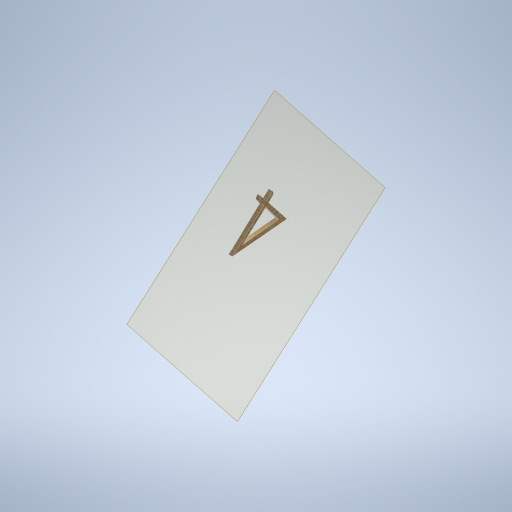
# Autodesk Inventor part: panel_block_03
Saved by Autodesk Inventor 2024.2 (Build 282272000, 272)
## iProperties
Created: 2024-05-21
Part Number: panel_block_03
Material: Wood (Maple)
Document SubType Name: Modeling
Designer: LOSTER_1
Density: 0.67 g/cm^3
Appearance: Natural Maple - Glossy Dark Tint
Author: LOSTER_1
Autodesk Inventor part; units mm, degrees
ref_plane "XZ Plane" through (0, 0, 0) normal (0, 1, 0) x (-1, 0, 0)
sketch "Sketch1" plane through (0, 0, 0) normal (0, 0, 1) x (1, 0, 0)
  arc A0 (4796.3585, -1909.6289) -> (3343.4744, 1121.5056) centre (-3903.1767, -4215.7265) ccw
  line L0 (3236.8192, 1046.7661) -> (3343.5051, 1121.464)
  arc A1 (3228.7635, 1285.3391) -> (1546.1726, 3076.3751) centre (-4110.5601, -3923.7232) ccw
  line L1 (3228.7635, 1285.3391) -> (3122.0787, 1210.6419)
  line L2 (1372.9503, 3176.3452) -> (1308.1705, 3064.1503)
  arc A2 (1372.9503, 3176.3452) -> (93.8576, 4024.2684) centre (-4221.2651, -3873.8147) ccw
  line L3 (1481.3729, 2964.1457) -> (1546.1726, 3076.3751)
  arc A3 (4543.4821, -2147.4888) -> (93.8528, 3844.2289) centre (-4256.4671, -4034.5221) ccw
  line L4 (93.8576, 4024.2684) -> (93.8528, 3844.2289)
  line L5 (1308.1705, 3064.1503) -> (1481.3729, 2964.1457)
  line L6 (3122.0787, 1210.6419) -> (3236.8192, 1046.7661)
  arc A4 (4543.4821, -2147.4888) -> (4796.3585, -1909.6289) centre (4134.8595, -1459.7188) ccw
  point P0 (0, 0)
  dimension "d7" = 800
  constraints: 14 end point, 11 point on circle, 5 centre point, 1 perpendicular
  measures "d7" radius of A4
ref_plane "Work Plane2" through (0, 0, -8101) normal (0, 0, 1) x (1, 0, 0)
ref_plane "Work Plane1" through (0, 0, 0) normal (0, 0, 1) x (1, 0, 0)
sketch "Sketch2" plane through (0, 0, -8101) normal (0, 0, 1) x (1, 0, 0)
  arc A0 (1192.0552, 3508.338) -> (93.8528, 4294.485) centre (-5164.5547, -4211.3454) ccw projected
  arc A1 (3133.8513, 1483.0798) -> (1365.2603, 3408.338) centre (-5051.6105, -4261.3276) ccw projected
  arc A2 (4543.6426, -2147.8414) -> (93.8528, 4114.0508) centre (-5207.4444, -4365.1147) ccw projected
  line L0 (1192.0552, 3508.338) -> (1126.9741, 3395.6142) projected
  line L1 (1365.2603, 3408.338) -> (1300.1792, 3295.6142) projected
  line L2 (1126.9741, 3395.6142) -> (1300.1792, 3295.6142) projected
  line L3 (93.8528, 4294.485) -> (93.8528, 4114.0508) projected
  line L4 (3027.6129, 1408.6909) -> (3133.8513, 1483.0798) projected
  line L5 (3142.3282, 1244.8605) -> (3248.5665, 1319.2494) projected
  line L6 (3027.6129, 1408.6909) -> (3142.3282, 1244.8605) projected
  arc A3 (4803.6655, -1899.2732) -> (3248.5665, 1319.2494) centre (-4832.968, -4570.4704) ccw projected
  arc A4 (4543.6426, -2147.8414) -> (4803.6655, -1899.2732) centre (4135.0016, -1460.0824) ccw projected
  point P0 (0, 0)
loft "Loft1" add profiles "Sketch1", "Sketch2"
ref_plane "Work Plane3" through (2600, 0, 0) normal (1, 0, 0) x (0, 1, 0)
sketch "Sketch3" plane through (2600, 0, 0) normal (1, 0, 0) x (0, 1, 0)
  line L0 (3120.8038, -3828.6818) -> (2179.9067, -2717.5683)
  line L1 (2179.9067, -2717.5683) -> (2281.1646, -4539.693)
  line L2 (2281.1646, -4539.693) -> (3120.8038, -3828.6818)
  line L3 (4534.6211, 332.5956) -> (-2270.5383, 332.5956)
  line L4 (-2270.5383, 332.5956) -> (-2270.5383, -8394.1003)
  line L5 (-2270.5383, -8394.1003) -> (4534.6211, -8394.1003)
  line L6 (4534.6211, -8394.1003) -> (4534.6211, 332.5956)
  point P0 (0, 0)
  constraints: 14 end point, 2 parallel, 2 perpendicular, 1 horizontal
extrude "Extrusion1" cut sketch "Sketch3" along normal through all both and the other way through all
sketch "Sketch5" plane through (2219.0112, 2281.1646, -4539.693) normal (0, -0.9984595, -0.0554857) x (1, 0, 0)
  line L0 (318.8718, 1824.936) -> (250.4195, 0)
  point P0 (-2219.0112, 4659.2715)
  constraints: 2 end point, 1 other
ref_plane "Work Plane4" through (2537.8831, 2179.9067, -2717.5683) normal (-0.6423359, -0.7662012, -0.0184479) x (-0.0374831, 0.0554467, -0.9977578)
sketch "Sketch6" plane through (2537.8831, 2179.9067, -2717.5683) normal (-0.6423359, -0.7662012, -0.0184479) x (-0.0374831, 0.0554467, -0.9977578)
  line L0 (-729.0595, -1938.3665) -> (2085.591, -1938.3665)
  line L1 (2085.591, -1938.3665) -> (2085.591, 179.9667)
  line L2 (2085.591, 179.9667) -> (-729.0595, 179.9667)
  line L3 (-729.0595, 179.9667) -> (-729.0595, -1938.3665)
  point P0 (-2737.216, -722.0143)
  constraints: 8 end point, 2 parallel, 1 horizontal, 1 perpendicular
extrude "Extrusion2" cut sketch "Sketch6" against normal through all
ref_plane "Work Plane5" through (2537.8831, 2179.9067, -2717.5683) normal (-0.9992973, -0.0020798, 0.0374254) x (-0.0374831, 0.0554467, -0.9977578)
sketch "Sketch7" plane through (2537.8831, 2179.9067, -2717.5683) normal (-0.9992973, -0.0020798, 0.0374254) x (-0.0374831, 0.0554467, -0.9977578)
  line L0 (1826.2193, 0) -> (0, 0) projected
  line L1 (1201.6643, -877.7967) -> (1826.2193, 0) projected
  line L2 (0, 0) -> (1201.6643, -877.7967) projected
  point P0 (-2737.216, 2025.7624)
sketch "Sketch8" plane through (2537.8831, 2179.9067, -2717.5683) normal (-0.6423359, -0.7662012, -0.0184479) x (-0.0374831, 0.0554467, -0.9977578)
  line L0 (1826.2193, 0) -> (0, 0) projected
  line L1 (1201.6643, -1365.6093) -> (1826.2193, 0) projected
  line L2 (0, 0) -> (1201.6643, -1365.6093) projected
  point P0 (-2737.216, -722.0143)
loft "Loft2" add profiles "Sketch7" section 1 edges at (2503.6569, 2230.5357, -3628.6306) (1958.4447, 2700.9842, -4184.1874) (1992.6709, 2650.3553, -3273.125)
sketch "Sketch9" plane through (2537.8831, 2179.9067, -2717.5683) normal (0.9992973, 0.0020798, -0.0374254) x (-0.0374831, 0.0554467, -0.9977578)
  line L0 (1201.6643, 877.7967) -> (0, 0) projected
  line L1 (1826.2193, 0) -> (0, 0) projected
  line L2 (1826.2193, 0) -> (1201.6643, 877.7967) projected
  point P0 (-2737.216, -2025.7624)
ref_plane "Work Plane6" through (2469.4307, 2281.1646, -4539.693) normal (0.9992973, 0.0020798, -0.0374254) x (0.0217303, 0.7814048, 0.623646)
sketch "Sketch10" plane through (2469.4307, 2281.1646, -4539.693) normal (0.9992973, 0.0020798, -0.0374254) x (0.0217303, 0.7814048, 0.623646)
  line L0 (1578.0672, -786.8916) -> (-983.5577, -786.8916)
  line L1 (-983.5577, -786.8916) -> (-983.5577, 1970.9014)
  line L2 (-983.5577, 1970.9014) -> (1578.0672, 1970.9014)
  line L3 (1578.0672, 1970.9014) -> (1578.0672, -786.8916)
  point P0 (994.987, 4892.7146)
  constraints: 8 end point, 2 parallel, 1 horizontal, 1 perpendicular
extrude "Extrusion3" cut sketch "Sketch10" against normal through all
sketch "Sketch11" plane through (2469.4307, 2281.1646, -4539.693) normal (0.9992973, 0.0020798, -0.0374254) x (0.0217303, 0.7814048, 0.623646)
  line L0 (1027.6784, 44.8475) -> (1011.4833, 1341.5246)
  line L1 (1011.4833, 1341.5246) -> (103.4312, 65.2798)
  line L2 (103.4312, 65.2798) -> (1027.6784, 44.8475)
  line L3 (960.9484, 1557.5799) -> (-216.8429, -97.7765)
  line L4 (960.9484, 1557.5799) -> (1128.2932, 1792.779)
  line L5 (1128.2932, 1585.7882) -> (1128.2932, 1792.779)
  line L6 (-69.5683, -97.7765) -> (-216.8429, -97.7765)
  line L7 (1027.6784, -97.7765) -> (1046.3487, -386.6685)
  line L8 (1182.7704, -360.1846) -> (1182.7704, -431.4012)
  arc A0 (1046.3487, -386.6685) -> (1182.7704, -431.4012) centre (1192.5364, -171.2284) ccw
  line L9 (1394.5704, -97.7765) -> (1471.9375, -97.7765)
  line L10 (1171.1456, 55.0636) -> (1464.8769, 44.8475)
  line L11 (1471.9375, -97.7765) -> (1528.8489, -97.7765)
  arc A1 (1528.8489, -97.7765) -> (1464.8769, 44.8475) centre (1251.9333, -136.3242) ccw
  line L12 (1128.2932, 1585.7882) -> (1171.1456, 55.0636)
  line L13 (1175.4243, -97.7765) -> (1182.7704, -360.1846)
  line L14 (-69.5683, -97.7765) -> (1027.6784, -97.7765)
  line L15 (1175.4243, -97.7765) -> (1394.5704, -97.7765)
  point P0 (994.987, 4892.7146)
  point P1 (1077.3097, 0)
  point P2 (1058.7249, 1488.0116)
  point P3 (0, 0)
  constraints: 32 end point, 4 point on circle, 3 horizontal, 2 centre point, 1 vertical
extrude "Extrusion4" add sketch "Sketch11" against normal blind 150
body "Solid1"
